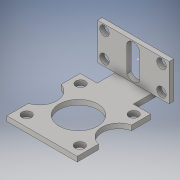
# Autodesk Inventor part: motor mount
Saved by Autodesk Inventor 2016 (Build 200138000, 138)
## iProperties
Created: 2017-09-14
Part Number: motor mount
Material: Generic
Document SubType Name: Modeling
Designer: student
Density: 1 g/cm^3
Appearance: Default
Author: student
Autodesk Inventor part; units mm, degrees
ref_plane "YZ Plane" through (0, 0, 0) normal (1, 0, 0) x (0, 1, 0)
ref_plane "XZ Plane" through (0, 0, 0) normal (0, 1, 0) x (-1, 0, 0)
ref_plane "XY Plane" through (0, 0, 0) normal (0, 0, 1) x (1, 0, 0)
sketch "Sketch1" plane through (0, 0, 0) normal (0, 0, 1) x (1, 0, 0)
  line L0 (-10.9855, -5.6515) -> (10.9855, -5.6515)
  line L1 (10.9855, -5.6515) -> (10.9855, 5.6515)
  line L2 (10.9855, 5.6515) -> (-10.9855, 5.6515)
  line L3 (-10.9855, 5.6515) -> (-10.9855, -5.6515)
  line L4 (-10.9855, -5.6515) -> (10.9855, 5.6515) construction
  line L5 (10.9855, -5.6515) -> (-10.9855, 5.6515) construction
  point P0 (0, 0)
  constraints: 12 end point, 2 midpoint, 2 parallel, 1 horizontal, 1 perpendicular
extrude "Extrusion1" add sketch "Sketch1" along normal blind 1.397
sketch "Sketch2" plane through (0, 0, 1.397) normal (0, 0, 1) x (1, 0, 0)
  circle A0 centre (-8.9011, 3.9017) radius 1.4605
  circle A1 centre (-8.9011, -3.6346) radius 1.4605
  circle A2 centre (8.6638, -3.6346) radius 1.4605
  circle A3 centre (8.6638, 3.9017) radius 1.4605
  line L0 (-2.0473, 3.9017) -> (-2.0473, -4.1687)
  line L1 (1.8989, 3.9017) -> (1.8989, -4.1687)
  arc A4 (1.8989, 3.9017) -> (-2.0473, 3.9017) centre (-0.0742, 3.3161) ccw
  arc A5 (-2.0473, -4.1687) -> (1.8989, -4.1687) centre (-0.0742, -3.0327) ccw
  point P0 (0, 0)
  constraints: 6 centre point, 4 end point, 4 point on circle, 2 vertical
extrude "Extrusion2" cut sketch "Sketch2" against normal blind 25.4
sketch "Sketch3" plane through (0, 0, 0) normal (0, 1, 0) x (-1, 0, 0)
  point P0 (0, 0)
sketch "Sketch4" plane through (0, 0, 1.397) normal (0, 0, 1) x (1, 0, 0)
  line L0 (-2.0473, -4.1687) -> (-5.6033, -4.1687)
  line L1 (1.9681, -4.1687) -> (5.5241, -4.1687)
  line L2 (-10.9855, -5.6515) -> (10.9855, -5.6515) projected
  line L3 (-5.6033, -5.6515) -> (5.5241, -5.6515)
  line L4 (5.5241, -5.6515) -> (5.5241, -7.4092)
  line L5 (5.5241, -7.4092) -> (-5.6033, -7.4092)
  line L6 (-5.6033, -7.4092) -> (-5.6033, -5.6515)
  point P0 (0, 0)
  dimension "d11" = 3.556
  dimension "d12" = 3.556
  constraints: 12 end point, 3 point on line, 2 horizontal, 2 parallel, 1 perpendicular
  measures "d11" distance of L0.start L0.end
  measures "d12" distance of L1.start L1.end
extrude "Extrusion3" add sketch "Sketch4" along normal blind 5.5626 and the other way blind 1.397
sketch "Sketch6" plane through (-5.6033, -5.6515, 1.397) normal (0, 1, 0) x (1, 0, 0)
  line L0 (-5.1994, -5.5615) -> (-5.1994, -11.4289)
  line L1 (16.4285, -5.5615) -> (16.4285, -11.4289)
  arc A0 (-5.1994, -21.5321) -> (-5.1994, -11.4289) centre (-6.7732, -16.4805) ccw
  arc A1 (16.4285, -11.4289) -> (16.4285, -21.5321) centre (17.5971, -16.4805) ccw
  line L2 (16.4285, -21.5321) -> (16.4285, -28.1107)
  line L3 (-5.1994, -21.5321) -> (-5.1994, -28.1107)
  line L4 (-5.1994, -28.1107) -> (16.4285, -28.1107)
  circle A2 centre (5.6145, -16.911) radius 5.9336
  circle A3 centre (-2.4076, -8.2492) radius 1.4605
  circle A4 centre (13.9302, -8.2492) radius 1.4605
  circle A5 centre (-2.4076, -24.8214) radius 1.4605
  circle A6 centre (13.9302, -24.8214) radius 1.4605
  line L5 (-5.1994, -5.5615) -> (16.4285, -5.5615)
  point P0 (5.6033, 1.397)
  dimension "d20" = 2.921
  dimension "d21" = 2.921
  dimension "d22" = 2.921
  dimension "d23" = 2.921
  constraints: 12 end point, 7 centre point, 4 point on circle, 4 vertical, 1 horizontal, 1 perpendicular
  measures "d20" diameter of A3
  measures "d21" diameter of A4
  measures "d22" diameter of A5
  measures "d23" diameter of A6
extrude "Extrusion4" add sketch "Sketch6" against normal blind 1.524
sketch "Sketch8" plane through (-5.6033, -7.4092, 6.9596) normal (0, -1, 0) x (1, 0, 0)
  line L0 (11.1274, -5.5626) -> (11.1274, -6.9596) projected
  line L1 (0, 0) -> (0, -6.9596) projected
  line L2 (11.1274, -6.9596) -> (0, -6.9596)
  line L3 (0, -6.9596) -> (0, 0)
  line L4 (0, 0) -> (11.1274, 0)
  line L5 (11.1274, 0) -> (11.1274, -6.9596)
  point P0 (5.6033, -6.9596)
  constraints: 8 end point, 2 parallel, 1 horizontal, 1 perpendicular
extrude "Extrusion5" cut sketch "Sketch8" against normal blind 0.2286
body "Solid1"
